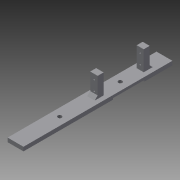
# Autodesk Inventor part: Top piece
Saved by Autodesk Inventor 2015 (Build 190159000, 159)
## iProperties
Created: 2014-11-22
Part Number: Top piece
Material: Generic
Document SubType Name: Modeling
Designer: jesse
Density: 1 g/cm^3
Appearance: Default
Author: jesse
Autodesk Inventor part; units mm, degrees
ref_plane "YZ Plane" through (0, 0, 0) normal (1, 0, 0) x (0, 1, 0)
ref_plane "XZ Plane" through (0, 0, 0) normal (0, 1, 0) x (-1, 0, 0)
ref_plane "XY Plane" through (0, 0, 0) normal (0, 0, 1) x (1, 0, 0)
sketch "Sketch1" plane through (0, 0, 0) normal (0, 0, 1) x (1, 0, 0)
  line L0 (10.1192, 6.6438) -> (35.5192, 6.6438)
  line L1 (35.5192, 6.6438) -> (35.5192, 0.2938)
  line L2 (35.5192, 0.2938) -> (10.1192, 0.2938)
  line L3 (10.1192, 0.2938) -> (10.1192, 6.6438)
  point P0 (0, 0)
  dimension "d0" = 25.4
  dimension "d1" = 6.35
  constraints: 8 end point, 2 parallel, 1 horizontal, 1 perpendicular
  measures "d0" distance of L1.end L2.end
  measures "d1" distance of L0.end L1.end
extrude "Extrusion1" add sketch "Sketch1" along normal blind 237.8075
sketch "Sketch2" plane through (10.1192, 6.6438, 0) normal (0, 1, 0) x (1, 0, 0)
  line L0 (0, 0) -> (25.4, 0) projected
  line L1 (0, 0) -> (0, -237.8075) projected
  line L2 (25.4, -237.8075) -> (0, -237.8075) projected
  line L3 (25.4, 0) -> (25.4, -237.8075) projected
  line L4 (12.7, 0) -> (12.7, -237.8075) construction
  line L5 (25.4, -237.8075) -> (0, -237.8075) construction
  line L6 (0, 0) -> (0, -237.8075) construction
  line L7 (0, -167.1637) -> (25.4, -167.1637) construction
  line L8 (0, -70.6437) -> (25.4, -70.6437) construction
  line L9 (25.4, 0) -> (25.4, -237.8075) construction
  circle A0 centre (12.7, -70.6437) radius 3.175
  circle A1 centre (12.7, -167.1637) radius 3.175
  line L10 (32.1721, -167.1637) -> (32.1721, -237.8075) construction
  line L11 (29.604, -70.6437) -> (29.604, 0) construction
  point P0 (-10.1192, 0)
  dimension "d6" = 6.35
  dimension "d7" = 6.35
  dimension "d10" = 96.52
  constraints: 10 end point, 8 point on line, 4 midpoint, 2 centre point, 2 parallel, 2 perpendicular, 1 vertical
  measures "d6" diameter of A0
  measures "d7" diameter of A1
  measures "d10" distance between parallel lines of L7 L8
extrude "Extrusion2" cut sketch "Sketch2" against normal through all contours A0 | A1
sketch "Sketch3" plane through (10.1192, 0.2938, 0) normal (-1, 0, 0) x (0, 0, 1)
  line L0 (44.8421, -2.7964) -> (94.9957, -2.7964)
  line L1 (94.9957, -2.7964) -> (94.9957, 2.2087)
  line L2 (94.9957, 2.2087) -> (44.8421, 2.2087)
  line L3 (44.8421, 2.2087) -> (44.8421, -2.7964)
  point P0 (0, -0.2938)
  constraints: 8 end point, 2 parallel, 1 horizontal, 1 perpendicular
extrude "Extrusion3" cut sketch "Sketch3" against normal through all
sketch "Sketch4" plane through (10.1192, 6.6438, 0) normal (0, 1, 0) x (1, 0, 0)
  line L0 (18.35, -38.735) -> (6.35, -38.735) projected
  line L1 (6.35, -102.735) -> (18.35, -102.735) projected
  line L2 (18.35, -38.735) -> (7.105, -38.735)
  line L3 (7.105, -38.735) -> (7.105, -29.21)
  line L4 (7.105, -29.21) -> (18.35, -29.21)
  line L5 (18.35, -29.21) -> (18.35, -38.735)
  line L6 (18.35, -102.735) -> (6.35, -102.735)
  line L7 (6.35, -102.735) -> (6.35, -112.26)
  line L8 (6.35, -112.26) -> (18.35, -112.26)
  line L9 (18.35, -112.26) -> (18.35, -102.735)
  point P0 (-10.1192, 0)
  dimension "d13" = 9.525
  dimension "d14" = 9.525
  constraints: 16 end point, 4 parallel, 2 horizontal, 2 perpendicular
  measures "d13" distance of L2.end L3.end
  measures "d14" distance of L7.end L6.end
extrude "Extrusion4" add sketch "Sketch4" along normal blind 30.1625
chamfer "Chamfer1" distance 4.7625 angle 45 2 edges at (22.8467, 6.6438, 29.21) (22.4692, 6.6438, 112.26)
sketch "Sketch5" plane through (16.4692, 36.8063, 112.26) normal (0, 0, 1) x (1, 0, 0)
  circle A0 centre (6, -22.1625) radius 1.3525 projected
  circle A1 centre (6, -6.1625) radius 1.3525 projected
  point P0 (-16.4692, -36.8063)
extrude "Extrusion5" cut sketch "Sketch5" against normal through all
fillet "Fillet1" radius 6.35 4 edges at (16.4692, 36.8063, 107.4975) (28.4692, 36.8063, 107.4975) (17.2242, 36.8063, 33.9725) (28.4692, 36.8063, 33.9725)
chamfer "Chamfer2" distance 4.7625 angle 45 4 edges at (16.4692, 6.6438, 109.8788) (28.4692, 6.6438, 109.8788) (28.4692, 6.6438, 31.5913) (17.2242, 6.6438, 31.5913)
body "Solid1"
